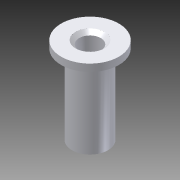
# Autodesk Inventor part: 13_0204_048
Saved by Autodesk Inventor 2012 SP1 (Build 160190100, 190)
## iProperties
Created: 2013-04-11
Part Number: 13_0204_048
Material: Default
Document SubType Name: Modeling
Designer: vogel
Density: 1 g/cm^3
Author: vogel
Autodesk Inventor part; units mm, degrees
ref_plane "YZ Plane" through (0, 0, 0) normal (1, 0, 0) x (0, 1, 0)
ref_plane "XZ Plane" through (0, 0, 0) normal (0, 1, 0) x (-1, 0, 0)
ref_plane "XY Plane" through (0, 0, 0) normal (0, 0, 1) x (1, 0, 0)
sketch "Skizze1" plane through (0, 0, 0) normal (0, 0, 1) x (1, 0, 0)
  circle A0 centre (0, 0) radius 2.5
  circle A1 centre (0, 0) radius 1.5
  dimension "d0" = 1
  dimension "d1" = 5
  constraints: 2 centre point, 2 coincident
  measures "d0" radial gap between concentric circles of A0 A1
  measures "d1" diameter of A0
extrude "Extrusion1" add sketch "Skizze1" along normal blind 12
chamfer "Fase1" distance 0.5 angle 45 2 edges at (-1.5, 0, 12) (-1.5, 0, 0)
sketch "Skizze2" plane through (0, 0, 12) normal (0, 0, 1) x (1, 0, 0)
  circle A0 centre (0, 0) radius 2.5 projected
  circle A1 centre (0, 0) radius 2 projected
  circle A2 centre (0, 0) radius 4
  dimension "d7" = 8
  constraints: 1 centre point, 1 coincident
  measures "d7" diameter of A2
extrude "Extrusion2" add sketch "Skizze2" against normal blind 1 contours A2
